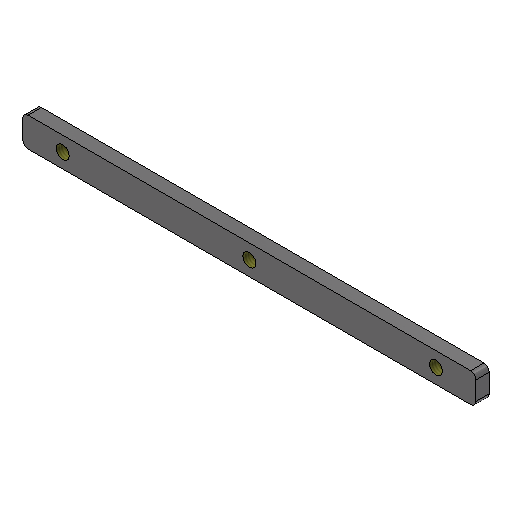
# Autodesk Inventor part: TL20240701-10120CV-017
Saved by Autodesk Inventor 2022.5 (Build 265521000, 521)
## iProperties
Category: FOLLOWER UNIT ASSY
Company: 현대 트랜시스(대유)
Created: 2023-04-10
Part Number: TL20240701-10120CV-017
Checked By: 김형민
Engr Approved By: 김시현
User Status: 2 x18
Material: SS400
Description: 0
Document SubType Name: Modeling
Mfg Approved By: 호상태
Designer: 박성규
Stock Number: 017
Density: 7.85 g/cm^3
Appearance: Plating Zinc White
Project: SW PJT
DETAIL: Coveryor Assembly
M/C TITLE: CJ 제일제당 협동로봇 포장시스탬 PILOT 장비
PARTS NAME: Bracket
SPECIFICATION: TA20221101-CV200000-015
DocNumber: 221118_Standard_v1
Folder: .\
VDS_Category: 엔지니어링
Detail Description: Processed products
Title: PLATE NUT
Subject: SW차종 시트조립라인
Author: 박성규
Revision Number: A
Autodesk Inventor part; units mm, degrees
ref_plane "YZ Plane" through (0, 0, 0) normal (1, 0, 0) x (0, 1, 0)
ref_plane "XZ Plane" through (0, 0, 0) normal (0, 1, 0) x (-1, 0, 0)
ref_plane "XY Plane" through (0, 0, 0) normal (0, 0, 1) x (1, 0, 0)
sketch "스케치9" plane through (0, 0, 0) normal (0, 0, 1) x (1, 0, 0)
  line L0 (-85, -5.5) -> (85, -5.5)
  line L1 (85, -5.5) -> (85, 5.5)
  line L2 (85, 5.5) -> (-85, 5.5)
  line L3 (-85, 5.5) -> (-85, -5.5)
  line L4 (-85, -5.5) -> (85, 5.5) construction
  line L5 (85, -5.5) -> (-85, 5.5) construction
  point P0 (0, 0)
  dimension "d40" = 170
  dimension "d41" = 11
  constraints: 12 end point, 2 midpoint, 2 parallel, 1 horizontal, 1 perpendicular
  measures "d40" distance of L1.end L2.end
  measures "d41" distance of L0.end L1.end
extrude "돌출4" add sketch "스케치9" along normal blind 5
fillet "모깎기2" radius 2 4 edges at (85, 5.5, 2.5) (85, -5.5, 2.5) (-85, 5.5, 2.5) (-85, -5.5, 2.5)
sketch "스케치10" plane through (0, 0, 5) normal (0, 0, 1) x (1, 0, 0)
  point P0 (0, 0)
  point P1 (0, 0)
  point P2 (-70, 0)
  point P3 (70, 0)
  dimension "d45" = 70
  dimension "d46" = 70
  constraints: 2 horizontal alignment, 1 coincident
  measures "d45" distance of point (0, 0) point (70, 0)
  measures "d46" distance of point (-70, 0) point (0, 0)
hole "구멍3" at (0, 0, 5) at (-70, 0, 5) at (70, 0, 5) direction (0, 0, -1) diameter 4.917 end through all thread size "M6x1" class "6H" standard "ISO Metric profile"
equation "\"d46\" = d45"
